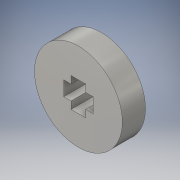
# Autodesk Inventor part: OmniShaft
Saved by Autodesk Inventor 2016 (Build 200138000, 138)
## iProperties
Created: 2017-02-08
Part Number: OmniShaft
Material: Generic
Document SubType Name: Modeling
Designer: Evan Phil George
Density: 1 g/cm^3
Appearance: Default
Author: Evan Phil George
Autodesk Inventor part; units mm, degrees
ref_plane "YZ Plane" through (0, 0, 0) normal (1, 0, 0) x (0, 1, 0)
ref_plane "XZ Plane" through (0, 0, 0) normal (0, 1, 0) x (-1, 0, 0)
ref_plane "XY Plane" through (0, 0, 0) normal (0, 0, 1) x (1, 0, 0)
sketch "Sketch1" plane through (0, 0, 0) normal (0, 0, 1) x (1, 0, 0)
  circle A0 centre (0, 0) radius 18
  dimension "d0" = 36
  constraints: 1 centre point, 1 coincident
  measures "d0" diameter of A0
extrude "Extrusion1" add sketch "Sketch1" along normal mid plane 9.5
sketch "Sketch2" plane through (0, 0, -4.75) normal (0, 0, -1) x (-1, 0, 0)
  line L0 (0, 0) -> (0, 6)
  line L1 (0, 6) -> (3, 6)
  line L2 (3, 6) -> (3, 3)
  line L3 (3, 3) -> (6, 3)
  line L4 (6, 3) -> (6, -3)
  line L5 (6, -3) -> (3, -3)
  line L6 (3, -3) -> (3, -6)
  line L7 (3, -6) -> (-3, -6)
  line L8 (-3, -6) -> (-3, -3)
  line L9 (-3, -3) -> (-6, -3)
  line L10 (-6, -3) -> (-6, 3)
  line L11 (-6, 3) -> (-3, 3)
  line L12 (-3, 3) -> (-3, 6)
  line L13 (-3, 6) -> (0, 6)
  dimension "d46" = 6
  dimension "d47" = 3
  dimension "d48" = 3
  dimension "d49" = 3
  dimension "d50" = 6
  dimension "d51" = 3
  dimension "d52" = 3
  dimension "d53" = 6
  dimension "d55" = 3
  dimension "d56" = 3
  dimension "d57" = 6
  dimension "d59" = 3
  dimension "d60" = 3
  constraints: 28 end point, 7 perpendicular, 2 horizontal, 2 point on line, 2 vertical
  measures "d46" distance of L0.start L0.end
  measures "d47" distance of L0.end L1.end
  measures "d48" distance of L1.end L2.end
  measures "d49" distance of L2.end L3.end
  measures "d50" distance of L3.end L4.end
  measures "d51" distance of L4.end L5.end
  measures "d52" distance of L5.end L6.end
  measures "d53" distance of L6.end L7.end
  measures "d55" distance of L7.end L8.end
  measures "d56" distance of L8.end L9.end
  measures "d57" distance of L9.end L10.end
  measures "d59" distance of L10.end L11.end
  measures "d60" distance of L11.end L12.end
extrude "Extrusion2" cut sketch "Sketch2" against normal blind 11
body "Solid1"
